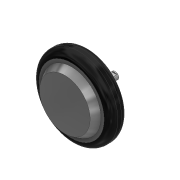
# Autodesk Inventor part: 10-001-ACTR
Saved by Autodesk Inventor 2018 (Build 220112000, 112)
## iProperties
Created: 2017-07-19
Part Number: 10-001-ACTR
Material: Aluminum 6061
Document SubType Name: Modeling
Designer: feesmrt
Density: 2.7 g/cm^3
Appearance: Aluminum - Polished
Author: feesmrt
Autodesk Inventor part; units mm, degrees
ref_plane "YZ Plane" through (0, 0, 0) normal (1, 0, 0) x (0, 1, 0)
ref_plane "XZ Plane" through (0, 0, 0) normal (0, 1, 0) x (-1, 0, 0)
ref_plane "XY Plane" through (0, 0, 0) normal (0, 0, 1) x (1, 0, 0)
sketch "Sketch1" plane through (0, 0, 0) normal (1, 0, 0) x (0, 1, 0)
  line L0 (0, 83.4) -> (0, -13.9) construction
  line L1 (-74.4, 0) -> (78.9, 0) construction
  line L2 (0, 69.5) -> (-38, 69.5)
  line L3 (-38, 69.5) -> (-38, 64)
  line L4 (-52.5, 55) -> (-52.5, 0)
  line L5 (-52.5, 55) -> (-38, 64)
  line L6 (-52.5, 0) -> (0, 0)
  line L7 (0, 69.5) -> (0, 15)
  line L8 (0, 15) -> (5, 10)
  line L9 (5, 10) -> (5, 7.95)
  line L10 (5, 7.95) -> (57, 7.95)
  line L11 (57, 7.95) -> (57, 0)
  line L12 (57, 0) -> (0, 0)
  dimension "d1" = 139
  dimension "d2" = 110
  dimension "d3" = 128
  dimension "d4" = 52.5
  dimension "d6" = 14.5
  dimension "d7" = 20
  dimension "d8" = 135
  dimension "d9" = 5
  dimension "d10" = 15.9
  dimension "d11" = 57
  constraints: 22 end point, 4 perpendicular, 4 point on line, 2 collinear, 2 horizontal
  measures "d1" diameter of L2 L1
  measures "d2" diameter of L4.start L1
  measures "d3" diameter of L3.end L1
  measures "d4" distance between parallel lines of L4 L0
  measures "d6" distance between parallel lines of L4 L3
  measures "d7" diameter of L8.end L1
  measures "d8" angle of L8 L9
  measures "d9" distance between parallel lines of L7 L9
  measures "d10" diameter of L10 L1
  measures "d11" distance between parallel lines of L7 L11
revolve "Base" add sketch "Sketch1" angle 360 about axis through (0, 0, 0) along (0, 1, 0)
sketch "Sketch2" plane through (0, 0, 0) normal (1, 0, 0) x (0, 1, 0)
  line L0 (5, 7.95) -> (57, 7.95) construction
  line L1 (5, -10) -> (5, 10) construction
  line L2 (57, -7.95) -> (57, 7.95) construction
  line L3 (10.5, 7.95) -> (10.5, 5.45)
  line L4 (10.5, 5.45) -> (54.5, 5.45)
  line L5 (54.5, 5.45) -> (54.5, 7.95)
  line L6 (5, -7.95) -> (57, -7.95) construction
  line L7 (10.5, 7.95) -> (54.5, 7.95)
  point P0 (0, 0)
  dimension "d13" = 13.4
  dimension "d14" = 5.5
  dimension "d15" = 2.5
  dimension "d16" = 44
  constraints: 8 end point, 3 perpendicular, 2 point on line, 1 collinear
  measures "d13" distance between parallel lines of L6 L4
  measures "d14" distance between parallel lines of L1 L3
  measures "d15" distance between parallel lines of L2 L5
  measures "d16" distance between parallel lines of L5 L3
extrude "Cut" cut sketch "Sketch2" along normal through all both and the other way through all
sketch "Sketch3" plane through (0, 0, 0) normal (1, 0, 0) x (0, 1, 0)
  line L0 (-38, 69.5) -> (0, 69.5) construction
  line L1 (-74.4, 0) -> (78.9, 0) construction
  line L2 (0, 97.3) -> (0, -97.3) construction
  line L3 (-38, -69.5) -> (-38, 69.5) construction
  line L4 (0, -69.5) -> (0, 69.5) projected
  line L5 (0, 69.5) -> (-38, 69.5)
  line L6 (-23, 86) -> (-15, 86)
  line L7 (-38, 69.5) -> (-38, 71)
  line L8 (0, 69.5) -> (0, 71)
  arc A0 (-23, 86) -> (-38, 71) centre (-23, 71) ccw
  arc A1 (0, 71) -> (-15, 86) centre (-15, 71) ccw
  point P0 (0, 0)
  point P1 (-38, 86)
  point P2 (0, 86)
  dimension "d21" = 172
  dimension "d22" = 15
  constraints: 8 end point, 5 point on line, 4 point on circle, 4 tangent, 2 centre point, 2 horizontal, 1 collinear, 1 equal radius, 1 vertical
  measures "d21" diameter of point (-38, 86) L1
  measures "d22" radius of A0
revolve "Revolution2" add sketch "Sketch3" angle 360 about axis through (0, 0, 0) along (0, 1, 0)
body "Solid1"
